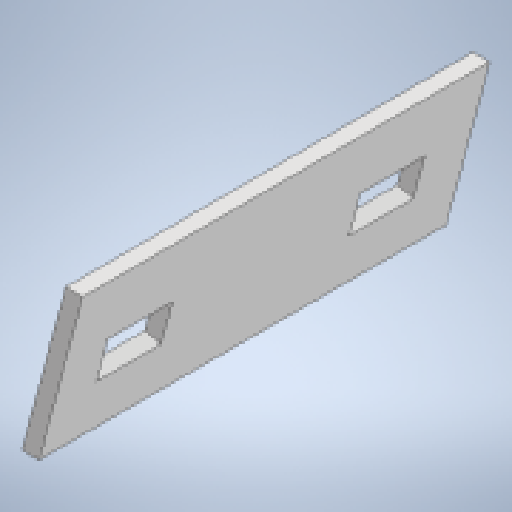
# Autodesk Inventor part: noz2
Saved by Autodesk Inventor 2023 (Build 270158000, 158)
## iProperties
Created: 2023-12-19
Part Number: noz2
Material: Ogólny
Document SubType Name: Modeling
Designer: Kamil
Density: 1 g/cm^3
Appearance: Domyślna
Author: Kamil
Autodesk Inventor part; units mm, degrees
ref_plane "YZ Plane" through (0, 0, 0) normal (1, 0, 0) x (0, 1, 0)
ref_plane "XZ Plane" through (0, 0, 0) normal (0, 1, 0) x (-1, 0, 0)
ref_plane "XY Plane" through (0, 0, 0) normal (0, 0, 1) x (1, 0, 0)
sketch "Szkic1" plane through (0, 0, 0) normal (0, 0, 1) x (1, 0, 0)
  line L0 (-10.5, 0) -> (0, 0) projected
  line L1 (0, 2) -> (-10.5, 2)
  line L2 (0, 2) -> (-5.359, -18)
  line L3 (-3.8837, -4.7669) -> (-2.0706, 2)
  line L4 (-3.8837, -4.7669) -> (-7.4295, -18)
  line L5 (-7.4295, -18) -> (-5.359, -18)
  dimension "d0" = 2
  dimension "d1" = 75
  dimension "d3" = 2
  dimension "d4" = 20
  constraints: 10 end point, 2 horizontal, 2 parallel, 1 point on line, 1 vertical alignment
  measures "d0" distance between parallel lines of L1 L0
  measures "d1" angle of L1 L2
  measures "d3" distance between parallel lines of L3 L2
  measures "d4" distance between parallel lines of L1 L5
extrude "Wyciągnięcie proste1" add sketch "Szkic1" against normal blind 50
sketch "Szkic2" plane through (-5.359, -18, 0) normal (0.9659258, -0.258819, 0) x (0, 0, -1)
  line L0 (42.7, 8.2894) -> (42.7, 10.6894) projected
  line L1 (38.3, 8.2894) -> (42.7, 8.2894) projected
  line L2 (7.3, 8.2894) -> (11.7, 8.2894) projected
  line L3 (11.7, 8.2894) -> (11.7, 10.6894) projected
  line L4 (42.7, 8.2894) -> (38.3, 8.2894)
  line L5 (38.3, 8.2894) -> (38.3, 10.6894)
  line L6 (38.3, 10.6894) -> (42.7, 10.6894)
  line L7 (42.7, 10.6894) -> (42.7, 8.2894)
  line L8 (11.7, 8.2894) -> (7.3, 8.2894)
  line L9 (7.3, 8.2894) -> (7.3, 10.6894)
  line L10 (7.3, 10.6894) -> (11.7, 10.6894)
  line L11 (11.7, 10.6894) -> (11.7, 8.2894)
  line L12 (43.7, 11.6894) -> (37.3, 11.6894)
  line L13 (37.3, 11.6894) -> (37.3, 7.2894)
  line L14 (37.3, 7.2894) -> (43.7, 7.2894)
  line L15 (43.7, 7.2894) -> (43.7, 11.6894)
  line L16 (12.7, 11.6894) -> (6.3, 11.6894)
  line L17 (6.3, 11.6894) -> (6.3, 7.2894)
  line L18 (6.3, 7.2894) -> (12.7, 7.2894)
  line L19 (12.7, 7.2894) -> (12.7, 11.6894)
  point P0 (0, 18.7737)
  dimension "d7" = 1
  dimension "d8" = 1
  constraints: 32 end point, 8 parallel, 4 perpendicular, 2 horizontal, 1 point on line, 6 other
  measures "d7" distance between parallel lines of L6 L12
  measures "d8" distance between parallel lines of L10 L16
extrude "Wyciągnięcie proste2" cut sketch "Szkic2" against normal through all contours L1 L5 L6 L0 | L9 L10 L3 L2 | L15 L14 L13 L12 | L19 L18 L17 L16
